Autodesk Fusion 360 part; units mm, degrees
note: some values were not read from the file. Set by a fixed rule: which face or edge a step refers to.
(part 12 of 13)
  spline S4 degree 5 poles (-1.3295, -6.4954) (-1.3295, -6.4955) (-1.3295, -6.4957) (-1.3296, -6.4961) (-1.3297, -6.4966) (-1.3299, -6.4975) (-1.33, -6.4984) (-1.3302, -6.4995) (-1.3304, -6.5007) (-1.3306, -6.502) (-1.3308, -6.5035) (-1.3311, -6.5051) (-1.3313, -6.5068) (-1.3316, -6.5086) (-1.3318, -6.5105) (-1.3321, -6.5126) (-1.3324, -6.5147) (-1.3326, -6.517) (-1.3329, -6.5194) (-1.3332, -6.5219) (-1.3335, -6.5245) (-1.3338, -6.5272) (-1.3341, -6.53) (-1.3343, -6.5329) (-1.3346, -6.5359) (-1.3349, -6.5391) (-1.3352, -6.5423) (-1.3354, -6.5456) (-1.3357, -6.549) (-1.3359, -6.5526) (-1.3362, -6.5562) (-1.3364, -6.5599) (-1.3366, -6.5637) (-1.3368, -6.5676) (-1.337, -6.5716) (-1.3372, -6.5757) (-1.3374, -6.5799) (-1.3376, -6.5842) (-1.3377, -6.5885) (-1.3379, -6.593) (-1.338, -6.5975) (-1.3381, -6.6021) (-1.3382, -6.6069) (-1.3383, -6.6117) (-1.3383, -6.6165) (-1.3384, -6.6215) (-1.3384, -6.6265) (-1.3384, -6.6317) (-1.3384, -6.6369) (-1.3383, -6.6422) (-1.3383, -6.6475) (-1.3382, -6.653) (-1.3381, -6.6585) (-1.338, -6.6641) (-1.3378, -6.6698) (-1.3376, -6.6755) (-1.3374, -6.6814) (-1.3372, -6.6873) (-1.337, -6.6933) (-1.3367, -6.6993) (-1.3364, -6.7054) (-1.3361, -6.7116) (-1.3357, -6.7179) (-1.3353, -6.7242) (-1.3349, -6.7306) (-1.3345, -6.7371) (-1.334, -6.7437) (-1.3335, -6.7503) (-1.333, -6.7569) (-1.3325, -6.7637) (-1.3319, -6.7705) (-1.3313, -6.7774) (-1.3306, -6.7843) (-1.3299, -6.7913) (-1.3292, -6.7984) (-1.3285, -6.8055) (-1.3277, -6.8127) (-1.3269, -6.82) (-1.3261, -6.8273) (-1.3252, -6.8347) (-1.3243, -6.8421) (-1.3234, -6.8496) (-1.3224, -6.8572) (-1.3214, -6.8648) (-1.3204, -6.8725) (-1.3193, -6.8802) (-1.3182, -6.888) (-1.317, -6.8958) (-1.3159, -6.9037) (-1.3146, -6.9117) (-1.3134, -6.9197) (-1.3121, -6.9278) (-1.3108, -6.9359) (-1.3094, -6.9441) (-1.308, -6.9523) (-1.3066, -6.9606) (-1.3051, -6.9689) (-1.3036, -6.9773) (-1.302, -6.9857) (-1.3004, -6.9942) (-1.2988, -7.0027) (-1.2971, -7.0113) (-1.2954, -7.0199) (-1.2936, -7.0286) (-1.2918, -7.0374) (-1.29, -7.0461) (-1.2881, -7.055) (-1.2862, -7.0638) (-1.2843, -7.0728) (-1.2823, -7.0817) (-1.2802, -7.0907) (-1.2782, -7.0998) (-1.276, -7.1089) (-1.2739, -7.118) (-1.2717, -7.1272) (-1.2694, -7.1365) (-1.2671, -7.1457) (-1.2648, -7.1551) (-1.2624, -7.1644) (-1.26, -7.1738) (-1.2575, -7.1833) (-1.255, -7.1928) (-1.2525, -7.2023) (-1.2499, -7.2118) (-1.2473, -7.2215) (-1.2446, -7.2311) (-1.2419, -7.2408) (-1.2391, -7.2505) (-1.2363, -7.2603) (-1.2334, -7.2701) (-1.2305, -7.2799) (-1.2276, -7.2898) (-1.2246, -7.2997) (-1.2215, -7.3096) (-1.2185, -7.3196) (-1.2153, -7.3296) (-1.2122, -7.3397) (-1.2089, -7.3498) (-1.2057, -7.3599) (-1.2024, -7.3701) (-1.199, -7.3803) (-1.1956, -7.3905) (-1.1922, -7.4007) (-1.1887, -7.411) (-1.1851, -7.4214) (-1.1815, -7.4317) (-1.1779, -7.4421) (-1.1742, -7.4525) (-1.1705, -7.463) (-1.1667, -7.4734) (-1.1629, -7.4839) (-1.159, -7.4945) (-1.1551, -7.5051) (-1.1511, -7.5157) (-1.1471, -7.5263) (-1.143, -7.5369) (-1.1389, -7.5476) (-1.1348, -7.5583) (-1.1306, -7.5691) (-1.1263, -7.5798) (-1.122, -7.5906) (-1.1176, -7.6014) (-1.1132, -7.6123) (-1.1088, -7.6232) (-1.1043, -7.6341) (-1.0997, -7.645) (-1.0951, -7.6559) (-1.0905, -7.6669) (-1.0858, -7.6779) (-1.0811, -7.6889) (-1.0763, -7.7) (-1.0714, -7.711) (-1.0665, -7.7221) (-1.0616, -7.7332) (-1.0566, -7.7444) (-1.0516, -7.7555) (-1.0465, -7.7667) (-1.0414, -7.7779) (-1.0362, -7.7891) (-1.0309, -7.8003) (-1.0256, -7.8116) (-1.0203, -7.8229) (-1.0149, -7.8342) (-1.0095, -7.8455) (-1.004, -7.8569) (-0.9985, -7.8682) (-0.9929, -7.8796) (-0.9872, -7.891) (-0.9815, -7.9024) (-0.9758, -7.9138) (-0.97, -7.9253) (-0.9642, -7.9368) (-0.9583, -7.9482) (-0.9524, -7.9597) (-0.9464, -7.9713) (-0.9403, -7.9828) (-0.9342, -7.9943) (-0.9281, -8.0059) (-0.9219, -8.0175) (-0.9157, -8.0291) (-0.9094, -8.0407) (-0.903, -8.0523) (-0.8966, -8.064) (-0.8902, -8.0756) (-0.8837, -8.0873) (-0.8771, -8.099) (-0.8705, -8.1107) (-0.8639, -8.1224) (-0.8572, -8.1341) (-0.8504, -8.1458) (-0.8436, -8.1575) (-0.8368, -8.1693) (-0.8299, -8.1811) (-0.8229, -8.1928) (-0.8159, -8.2046) (-0.8089, -8.2164) (-0.8018, -8.2282) (-0.7946, -8.2401) (-0.7874, -8.2519) (-0.7801, -8.2637) (-0.7728, -8.2756) (-0.7655, -8.2874) (-0.758, -8.2993) (-0.7506, -8.3112) (-0.743, -8.3231) (-0.7355, -8.3349) (-0.7279, -8.3468) (-0.7202, -8.3587) (-0.7125, -8.3707) (-0.7047, -8.3826) (-0.6969, -8.3945) (-0.689, -8.4064) (-0.6811, -8.4184) (-0.6731, -8.4303) (-0.665, -8.4423) (-0.657, -8.4542) (-0.6488, -8.4662) (-0.6406, -8.4782) (-0.6324, -8.4901) (-0.6241, -8.5021) (-0.6158, -8.5141) (-0.6091, -8.5237) (-0.604, -8.5309) (-0.6006, -8.5357) (-0.5989, -8.5381) knots 0 0 0 0 0 0 0.00416667 0.00833333 0.0125 0.01666667 0.02083333 0.025 0.02916667 0.03333333 0.0375 0.04166667 0.04583333 0.05 0.05416667 0.05833333 0.0625 0.06666667 0.07083333 0.075 0.07916667 0.08333333 0.0875 0.09166667 0.09583333 0.1 0.10416667 0.10833333 0.1125 0.11666667 0.12083333 0.125 0.12916667 0.13333333 0.1375 0.14166667 0.14583333 0.15 0.15416667 0.15833333 0.1625 0.16666667 0.17083333 0.175 0.17916667 0.18333333 0.1875 0.19166667 0.19583333 0.2 0.20416667 0.20833333 0.2125 0.21666667 0.22083333 0.225 0.22916667 0.23333333 0.2375 0.24166667 0.24583333 0.25 0.25416667 0.25833333 0.2625 0.26666667 0.27083333 0.275 0.27916667 0.28333333 0.2875 0.29166667 0.29583333 0.3 0.30416667 0.30833333 0.3125 0.31666667 0.32083333 0.325 0.32916667 0.33333333 0.3375 0.34166667 0.34583333 0.35 0.35416667 0.35833333 0.3625 0.36666667 0.37083333 0.375 0.37916667 0.38333333 0.3875 0.39166667 0.39583333 0.4 0.40416667 0.40833333 0.4125 0.41666667 0.42083333 0.425 0.42916667 0.43333333 0.4375 0.44166667 0.44583333 0.45 0.45416667 0.45833333 0.4625 0.46666667 0.47083333 0.475 0.47916667 0.48333333 0.4875 0.49166667 0.49583333 0.5 0.50416667 0.50833333 0.5125 0.51666667 0.52083333 0.525 0.52916667 0.53333333 0.5375 0.54166667 0.54583333 0.55 0.55416667 0.55833333 0.5625 0.56666667 0.57083333 0.575 0.57916667 0.58333333 0.5875 0.59166667 0.59583333 0.6 0.60416667 0.60833333 0.6125 0.61666667 0.62083333 0.625 0.62916667 0.63333333 0.6375 0.64166667 0.64583333 0.65 0.65416667 0.65833333 0.6625 0.66666667 0.67083333 0.675 0.67916667 0.68333333 0.6875 0.69166667 0.69583333 0.7 0.70416667 0.70833333 0.7125 0.71666667 0.72083333 0.725 0.72916667 0.73333333 0.7375 0.74166667 0.74583333 0.75 0.75416667 0.75833333 0.7625 0.76666667 0.77083333 0.775 0.77916667 0.78333333 0.7875 0.79166667 0.79583333 0.8 0.80416667 0.80833333 0.8125 0.81666667 0.82083333 0.825 0.82916667 0.83333333 0.8375 0.84166667 0.84583333 0.85 0.85416667 0.85833333 0.8625 0.86666667 0.87083333 0.875 0.87916667 0.88333333 0.8875 0.89166667 0.89583333 0.9 0.90416667 0.90833333 0.9125 0.91666667 0.92083333 0.925 0.92916667 0.93333333 0.9375 0.94166667 0.94583333 0.95 0.95416667 0.95833333 0.9625 0.96666667 0.97083333 0.975 0.97916667 0.98333333 0.9875 0.99166667 0.99583333 1 1 1 1 1 1
  arc A5 (-0.5989, -8.5381) -> (0.5989, -8.5381) centre (0, 0) ccw
  spline S5 degree 5 poles (0.5989, -8.5381) (0.6006, -8.5357) (0.604, -8.5309) (0.6091, -8.5237) (0.6158, -8.5141) (0.6241, -8.5021) (0.6324, -8.4901) (0.6406, -8.4782) (0.6488, -8.4662) (0.657, -8.4542) (0.665, -8.4423) (0.6731, -8.4303) (0.6811, -8.4184) (0.689, -8.4064) (0.6969, -8.3945) (0.7047, -8.3826) (0.7125, -8.3707) (0.7202, -8.3587) (0.7279, -8.3468) (0.7355, -8.3349) (0.743, -8.3231) (0.7506, -8.3112) (0.758, -8.2993) (0.7655, -8.2874) (0.7728, -8.2756) (0.7801, -8.2637) (0.7874, -8.2519) (0.7946, -8.2401) (0.8018, -8.2282) (0.8089, -8.2164) (0.8159, -8.2046) (0.8229, -8.1928) (0.8299, -8.1811) (0.8368, -8.1693) (0.8436, -8.1575) (0.8504, -8.1458) (0.8572, -8.1341) (0.8639, -8.1224) (0.8705, -8.1107) (0.8771, -8.099) (0.8837, -8.0873) (0.8902, -8.0756) (0.8966, -8.064) (0.903, -8.0523) (0.9094, -8.0407) (0.9157, -8.0291) (0.9219, -8.0175) (0.9281, -8.0059) (0.9342, -7.9943) (0.9403, -7.9828) (0.9464, -7.9713) (0.9524, -7.9597) (0.9583, -7.9482) (0.9642, -7.9368) (0.97, -7.9253) (0.9758, -7.9138) (0.9815, -7.9024) (0.9872, -7.891) (0.9929, -7.8796) (0.9985, -7.8682) (1.004, -7.8569) (1.0095, -7.8455) (1.0149, -7.8342) (1.0203, -7.8229) (1.0256, -7.8116) (1.0309, -7.8003) (1.0362, -7.7891) (1.0414, -7.7779) (1.0465, -7.7667) (1.0516, -7.7555) (1.0566, -7.7444) (1.0616, -7.7332) (1.0665, -7.7221) (1.0714, -7.711) (1.0763, -7.7) (1.0811, -7.6889) (1.0858, -7.6779) (1.0905, -7.6669) (1.0951, -7.6559) (1.0997, -7.645) (1.1043, -7.6341) (1.1088, -7.6232) (1.1132, -7.6123) (1.1176, -7.6014) (1.122, -7.5906) (1.1263, -7.5798) (1.1306, -7.5691) (1.1348, -7.5583) (1.1389, -7.5476) (1.143, -7.5369) (1.1471, -7.5263) (1.1511, -7.5157) (1.1551, -7.5051) (1.159, -7.4945) (1.1629, -7.4839) (1.1667, -7.4734) (1.1705, -7.463) (1.1742, -7.4525) (1.1779, -7.4421) (1.1815, -7.4317) (1.1851, -7.4214) (1.1887, -7.411) (1.1922, -7.4007) (1.1956, -7.3905) (1.199, -7.3803) (1.2024, -7.3701) (1.2057, -7.3599) (1.2089, -7.3498) (1.2122, -7.3397) (1.2153, -7.3296) (1.2185, -7.3196) (1.2215, -7.3096) (1.2246, -7.2997) (1.2276, -7.2898) (1.2305, -7.2799) (1.2334, -7.2701) (1.2363, -7.2603) (1.2391, -7.2505) (1.2419, -7.2408) (1.2446, -7.2311) (1.2473, -7.2215) (1.2499, -7.2118) (1.2525, -7.2023) (1.255, -7.1928) (1.2575, -7.1833) (1.26, -7.1738) (1.2624, -7.1644) (1.2648, -7.1551) (1.2671, -7.1457) (1.2694, -7.1365) (1.2717, -7.1272) (1.2739, -7.118) (1.276, -7.1089) (1.2782, -7.0998) (1.2802, -7.0907) (1.2823, -7.0817) (1.2843, -7.0728) (1.2862, -7.0638) (1.2881, -7.055) (1.29, -7.0461) (1.2918, -7.0374) (1.2936, -7.0286) (1.2954, -7.0199) (1.2971, -7.0113) (1.2988, -7.0027) (1.3004, -6.9942) (1.302, -6.9857) (1.3036, -6.9773) (1.3051, -6.9689) (1.3066, -6.9606) (1.308, -6.9523) (1.3094, -6.9441) (1.3108, -6.9359) (1.3121, -6.9278) (1.3134, -6.9197) (1.3146, -6.9117) (1.3159, -6.9037) (1.317, -6.8958) (1.3182, -6.888) (1.3193, -6.8802) (1.3204, -6.8725) (1.3214, -6.8648) (1.3224, -6.8572) (1.3234, -6.8496) (1.3243, -6.8421) (1.3252, -6.8347) (1.3261, -6.8273) (1.3269, -6.82) (1.3277, -6.8127) (1.3285, -6.8055) (1.3292, -6.7984) (1.3299, -6.7913) (1.3306, -6.7843) (1.3313, -6.7774) (1.3319, -6.7705) (1.3325, -6.7637) (1.333, -6.7569) (1.3335, -6.7503) (1.334, -6.7437) (1.3345, -6.7371) (1.3349, -6.7306) (1.3353, -6.7242) (1.3357, -6.7179) (1.3361, -6.7116) (1.3364, -6.7054) (1.3367, -6.6993) (1.337, -6.6933) (1.3372, -6.6873) (1.3374, -6.6814) (1.3376, -6.6755) (1.3378, -6.6698) (1.338, -6.6641) (1.3381, -6.6585) (1.3382, -6.653) (1.3383, -6.6475) (1.3383, -6.6422) (1.3384, -6.6369) (1.3384, -6.6317) (1.3384, -6.6265) (1.3384, -6.6215) (1.3383, -6.6165) (1.3383, -6.6117) (1.3382, -6.6069) (1.3381, -6.6021) (1.338, -6.5975) (1.3379, -6.593) (1.3377, -6.5885) (1.3376, -6.5842) (1.3374, -6.5799) (1.3372, -6.5757) (1.337, -6.5716) (1.3368, -6.5676) (1.3366, -6.5637) (1.3364, -6.5599) (1.3362, -6.5562) (1.3359, -6.5526) (1.3357, -6.549) (1.3354, -6.5456) (1.3352, -6.5423) (1.3349, -6.5391) (1.3346, -6.5359) (1.3343, -6.5329) (1.3341, -6.53) (1.3338, -6.5272) (1.3335, -6.5245) (1.3332, -6.5219) (1.3329, -6.5194) (1.3326, -6.517) (1.3324, -6.5147) (1.3321, -6.5126) (1.3318, -6.5105) (1.3316, -6.5086) (1.3313, -6.5068) (1.3311, -6.5051) (1.3308, -6.5035) (1.3306, -6.502) (1.3304, -6.5007) (1.3302, -6.4995) (1.33, -6.4984) (1.3299, -6.4975) (1.3297, -6.4966) (1.3296, -6.4961) (1.3295, -6.4957) (1.3295, -6.4955) (1.3295, -6.4954) knots -1 -1 -1 -1 -1 -1 -0.99583333 -0.99166667 -0.9875 -0.98333333 -0.97916667 -0.975 -0.97083333 -0.96666667 -0.9625 -0.95833333 -0.95416667 -0.95 -0.94583333 -0.94166667 -0.9375 -0.93333333 -0.92916667 -0.925 -0.92083333 -0.91666667 -0.9125 -0.90833333 -0.90416667 -0.9 -0.89583333 -0.89166667 -0.8875 -0.88333333 -0.87916667 -0.875 -0.87083333 -0.86666667 -0.8625 -0.85833333 -0.85416667 -0.85 -0.84583333 -0.84166667 -0.8375 -0.83333333 -0.82916667 -0.825 -0.82083333 -0.81666667 -0.8125 -0.80833333 -0.80416667 -0.8 -0.79583333 -0.79166667 -0.7875 -0.78333333 -0.77916667 -0.775 -0.77083333 -0.76666667 -0.7625 -0.75833333 -0.75416667 -0.75 -0.74583333 -0.74166667 -0.7375 -0.73333333 -0.72916667 -0.725 -0.72083333 -0.71666667 -0.7125 -0.70833333 -0.70416667 -0.7 -0.69583333 -0.69166667 -0.6875 -0.68333333 -0.67916667 -0.675 -0.67083333 -0.66666667 -0.6625 -0.65833333 -0.65416667 -0.65 -0.64583333 -0.64166667 -0.6375 -0.63333333 -0.62916667 -0.625 -0.62083333 -0.61666667 -0.6125 -0.60833333 -0.60416667 -0.6 -0.59583333 -0.59166667 -0.5875 -0.58333333 -0.57916667 -0.575 -0.57083333 -0.56666667 -0.5625 -0.55833333 -0.55416667 -0.55 -0.54583333 -0.54166667 -0.5375 -0.53333333 -0.52916667 -0.525 -0.52083333 -0.51666667 -0.5125 -0.50833333 -0.50416667 -0.5 -0.49583333 -0.49166667 -0.4875 -0.48333333 -0.47916667 -0.475 -0.47083333 -0.46666667 -0.4625 -0.45833333 -0.45416667 -0.45 -0.44583333 -0.44166667 -0.4375 -0.43333333 -0.42916667 -0.425 -0.42083333 -0.41666667 -0.4125 -0.40833333 -0.40416667 -0.4 -0.39583333 -0.39166667 -0.3875 -0.38333333 -0.37916667 -0.375 -0.37083333 -0.36666667 -0.3625 -0.35833333 -0.35416667 -0.35 -0.34583333 -0.34166667 -0.3375 -0.33333333 -0.32916667 -0.325 -0.32083333 -0.31666667 -0.3125 -0.30833333 -0.30416667 -0.3 -0.29583333 -0.29166667 -0.2875 -0.28333333 -0.27916667 -0.275 -0.27083333 -0.26666667 -0.2625 -0.25833333 -0.25416667 -0.25 -0.24583333 -0.24166667 -0.2375 -0.23333333 -0.22916667 -0.225 -0.22083333 -0.21666667 -0.2125 -0.20833333 -0.20416667 -0.2 -0.19583333 -0.19166667 -0.1875 -0.18333333 -0.17916667 -0.175 -0.17083333 -0.16666667 -0.1625 -0.15833333 -0.15416667 -0.15 -0.14583333 -0.14166667 -0.1375 -0.13333333 -0.12916667 -0.125 -0.12083333 -0.11666667 -0.1125 -0.10833333 -0.10416667 -0.1 -0.09583333 -0.09166667 -0.0875 -0.08333333 -0.07916667 -0.075 -0.07083333 -0.06666667 -0.0625 -0.05833333 -0.05416667 -0.05 -0.04583333 -0.04166667 -0.0375 -0.03333333 -0.02916667 -0.025 -0.02083333 -0.01666667 -0.0125 -0.00833333 -0.00416667 0 0 0 0 0 0
  line L10 (1.3295, -6.4954) -> (1.3293, -6.4945)
  line L11 (1.3293, -6.4945) -> (0.944, -4.6119)
  arc A6 (0.944, -4.6119) -> (2.5936, -3.9286) centre (0, 0) ccw
  line L12 (2.5936, -3.9286) -> (3.6523, -5.5323)
  line L13 (3.6523, -5.5323) -> (3.6529, -5.533)
  spline S6 degree 5 poles (3.6529, -5.533) (3.6529, -5.5331) (3.653, -5.5333) (3.6532, -5.5336) (3.6536, -5.5341) (3.654, -5.5348) (3.6546, -5.5355) (3.6552, -5.5364) (3.656, -5.5374) (3.6568, -5.5385) (3.6576, -5.5397) (3.6586, -5.541) (3.6596, -5.5424) (3.6607, -5.5438) (3.6619, -5.5454) (3.6632, -5.547) (3.6645, -5.5487) (3.6659, -5.5505) (3.6674, -5.5524) (3.6689, -5.5544) (3.6706, -5.5564) (3.6723, -5.5585) (3.6741, -5.5607) (3.676, -5.563) (3.6779, -5.5653) (3.6799, -5.5677) (3.682, -5.5702) (3.6842, -5.5727) (3.6864, -5.5753) (3.6887, -5.578) (3.6911, -5.5807) (3.6936, -5.5835) (3.6961, -5.5864) (3.6987, -5.5893) (3.7014, -5.5923) (3.7042, -5.5953) (3.707, -5.5984) (3.7099, -5.6015) (3.7129, -5.6047) (3.7159, -5.608) (3.719, -5.6113) (3.7222, -5.6146) (3.7255, -5.618) (3.7288, -5.6214) (3.7323, -5.6249) (3.7357, -5.6285) (3.7393, -5.6321) (3.7429, -5.6357) (3.7466, -5.6394) (3.7504, -5.6431) (3.7542, -5.6468) (3.7581, -5.6506) (3.7621, -5.6544) (3.7662, -5.6583) (3.7703, -5.6622) (3.7745, -5.6662) (3.7787, -5.6702) (3.7831, -5.6742) (3.7875, -5.6782) (3.7919, -5.6823) (3.7965, -5.6864) (3.8011, -5.6906) (3.8058, -5.6948) (3.8105, -5.699) (3.8153, -5.7032) (3.8202, -5.7075) (3.8252, -5.7118) (3.8302, -5.7161) (3.8353, -5.7205) (3.8405, -5.7248) (3.8457, -5.7292) (3.851, -5.7337) (3.8563, -5.7381) (3.8618, -5.7426) (3.8673, -5.7471) (3.8728, -5.7516) (3.8785, -5.7562) (3.8842, -5.7607) (3.8899, -5.7653) (3.8958, -5.7699) (3.9017, -5.7745) (3.9076, -5.7792) (3.9137, -5.7838) (3.9198, -5.7885) (3.9259, -5.7932) (3.9321, -5.7979) (3.9384, -5.8026) (3.9448, -5.8074) (3.9512, -5.8121) (3.9577, -5.8169) (3.9643, -5.8217) (3.9709, -5.8265) (3.9776, -5.8313) (3.9843, -5.8361) (3.9911, -5.8409) (3.998, -5.8457) (4.0049, -5.8506) (4.0119, -5.8554) (4.019, -5.8603) (4.0261, -5.8652) (4.0333, -5.8701) (4.0406, -5.8749) (4.0479, -5.8798) (4.0553, -5.8847) (4.0627, -5.8896) (4.0702, -5.8945) (4.0778, -5.8995) (4.0854, -5.9044) (4.0931, -5.9093) (4.1008, -5.9142) (4.1086, -5.9192) (4.1165, -5.9241) (4.1245, -5.929) (4.1325, -5.934) (4.1405, -5.9389) (4.1486, -5.9439) (4.1568, -5.9488) (4.165, -5.9537) (4.1733, -5.9587) (4.1817, -5.9636) (4.1901, -5.9686) (4.1986, -5.9735) (4.2071, -5.9784) (4.2157, -5.9834) (4.2244, -5.9883) (4.2331, -5.9932) (4.2419, -5.9981) (4.2507, -6.0031) (4.2596, -6.008) (4.2686, -6.0129) (4.2776, -6.0178) (4.2866, -6.0227) (4.2958, -6.0276) (4.3049, -6.0325) (4.3142, -6.0373) (4.3235, -6.0422) (4.3328, -6.0471) (4.3422, -6.0519) (4.3517, -6.0568) (4.3612, -6.0616) (4.3708, -6.0665) (4.3804, -6.0713) (4.3901, -6.0761) (4.3999, -6.0809) (4.4097, -6.0857) (4.4195, -6.0905) (4.4295, -6.0952) (4.4394, -6.1) (4.4495, -6.1048) (4.4595, -6.1095) (4.4697, -6.1142) (4.4799, -6.1189) (4.4901, -6.1236) (4.5004, -6.1283) (4.5108, -6.133) (4.5212, -6.1377) (4.5316, -6.1423) (4.5421, -6.1469) (4.5527, -6.1516) (4.5633, -6.1562) (4.574, -6.1607) (4.5847, -6.1653) (4.5955, -6.1699) (4.6064, -6.1744) (4.6172, -6.1789) (4.6282, -6.1835) (4.6392, -6.1879) (4.6502, -6.1924) (4.6613, -6.1969) (4.6725, -6.2013) (4.6836, -6.2057) (4.6949, -6.2101) (4.7062, -6.2145) (4.7175, -6.2189) (4.7289, -6.2232) (4.7404, -6.2275) (4.7519, -6.2319) (4.7634, -6.2361) (4.7751, -6.2404) (4.7867, -6.2447) (4.7984, -6.2489) (4.8102, -6.2531) (4.822, -6.2573) (4.8338, -6.2614) (4.8457, -6.2656) (4.8577, -6.2697) (4.8696, -6.2738) (4.8817, -6.2779) (4.8938, -6.2819) (4.9059, -6.2859) (4.9181, -6.2899) (4.9304, -6.2939) (4.9426, -6.2979) (4.955, -6.3018) (4.9673, -6.3057) (4.9798, -6.3096) (4.9922, -6.3135) (5.0048, -6.3173) (5.0173, -6.3211) (5.0299, -6.3249) (5.0426, -6.3287) (5.0553, -6.3324) (5.0681, -6.3361) (5.0809, -6.3398) (5.0937, -6.3434) (5.1066, -6.3471) (5.1195, -6.3507) (5.1325, -6.3542) (5.1455, -6.3578) (5.1586, -6.3613) (5.1717, -6.3648) (5.1849, -6.3683) (5.1981, -6.3717) (5.2113, -6.3751) (5.2246, -6.3785) (5.2379, -6.3819) (5.2513, -6.3852) (5.2647, -6.3885) (5.2782, -6.3917) (5.2917, -6.395) (5.3053, -6.3982) (5.3188, -6.4014) (5.3325, -6.4045) (5.3462, -6.4076) (5.3599, -6.4107) (5.3736, -6.4138) (5.3874, -6.4168) (5.4013, -6.4198) (5.4152, -6.4227) (5.4291, -6.4257) (5.4431, -6.4286) (5.4571, -6.4314) (5.4711, -6.4343) (5.4852, -6.4371) (5.4993, -6.4399) (5.5135, -6.4426) (5.5277, -6.4453) (5.542, -6.448) (5.5563, -6.4506) (5.5706, -6.4532) (5.585, -6.4558) (5.5965, -6.4578) (5.6051, -6.4593) (5.6109, -6.4603) (5.6138, -6.4608) knots 0 0 0 0 0 0 0.00416667 0.00833333 0.0125 0.01666667 0.02083333 0.025 0.02916667 0.03333333 0.0375 0.04166667 0.04583333 0.05 0.05416667 0.05833333 0.0625 0.06666667 0.07083333 0.075 0.07916667 0.08333333 0.0875 0.09166667 0.09583333 0.1 0.10416667 0.10833333 0.1125 0.11666667 0.12083333 0.125 0.12916667 0.13333333 0.1375 0.14166667 0.14583333 0.15 0.15416667 0.15833333 0.1625 0.16666667 0.17083333 0.175 0.17916667 0.18333333 0.1875 0.19166667 0.19583333 0.2 0.20416667 0.20833333 0.2125 0.21666667 0.22083333 0.225 0.22916667 0.23333333 0.2375 0.24166667 0.24583333 0.25 0.25416667 0.25833333 0.2625 0.26666667 0.27083333 0.275 0.27916667 0.28333333 0.2875 0.29166667 0.29583333 0.3 0.30416667 0.30833333 0.3125 0.31666667 0.32083333 0.325 0.32916667 0.33333333 0.3375 0.34166667 0.34583333 0.35 0.35416667 0.35833333 0.3625 0.36666667 0.37083333 0.375 0.37916667 0.38333333 0.3875 0.39166667 0.39583333 0.4 0.40416667 0.40833333 0.4125 0.41666667 0.42083333 0.425 0.42916667 0.43333333 0.4375 0.44166667 0.44583333 0.45 0.45416667 0.45833333 0.4625 0.46666667 0.47083333 0.475 0.47916667 0.48333333 0.4875 0.49166667 0.49583333 0.5 0.50416667 0.50833333 0.5125 0.51666667 0.52083333 0.525 0.52916667 0.53333333 0.5375 0.54166667 0.54583333 0.55 0.55416667 0.55833333 0.5625 0.56666667 0.57083333 0.575 0.57916667 0.58333333 0.5875 0.59166667 0.59583333 0.6 0.60416667 0.60833333 0.6125 0.61666667 0.62083333 0.625 0.62916667 0.63333333 0.6375 0.64166667 0.64583333 0.65 0.65416667 0.65833333 0.6625 0.66666667 0.67083333 0.675 0.67916667 0.68333333 0.6875 0.69166667 0.69583333 0.7 0.70416667 0.70833333 0.7125 0.71666667 0.72083333 0.725 0.72916667 0.73333333 0.7375 0.74166667 0.74583333 0.75 0.75416667 0.75833333 0.7625 0.76666667 0.77083333 0.775 0.77916667 0.78333333 0.7875 0.79166667 0.79583333 0.8 0.80416667 0.80833333 0.8125 0.81666667 0.82083333 0.825 0.82916667 0.83333333 0.8375 0.84166667 0.84583333 0.85 0.85416667 0.85833333 0.8625 0.86666667 0.87083333 0.875 0.87916667 0.88333333 0.8875 0.89166667 0.89583333 0.9 0.90416667 0.90833333 0.9125 0.91666667 0.92083333 0.925 0.92916667 0.93333333 0.9375 0.94166667 0.94583333 0.95 0.95416667 0.95833333 0.9625 0.96666667 0.97083333 0.975 0.97916667 0.98333333 0.9875 0.99166667 0.99583333 1 1 1 1 1 1
  arc A7 (5.6138, -6.4608) -> (6.4608, -5.6138) centre (0, 0) ccw
  spline S7 degree 5 poles (6.4608, -5.6138) (6.4603, -5.6109) (6.4593, -5.6051) (6.4578, -5.5965) (6.4558, -5.585) (6.4532, -5.5706) (6.4506, -5.5563) (6.448, -5.542) (6.4453, -5.5277) (6.4426, -5.5135) (6.4399, -5.4993) (6.4371, -5.4852) (6.4343, -5.4711) (6.4314, -5.4571) (6.4286, -5.4431) (6.4257, -5.4291) (6.4227, -5.4152) (6.4198, -5.4013) (6.4168, -5.3874) (6.4138, -5.3736) (6.4107, -5.3599) (6.4076, -5.3462) (6.4045, -5.3325) (6.4014, -5.3188) (6.3982, -5.3053) (6.395, -5.2917) (6.3917, -5.2782) (6.3885, -5.2647) (6.3852, -5.2513) (6.3819, -5.2379) (6.3785, -5.2246) (6.3751, -5.2113) (6.3717, -5.1981) (6.3683, -5.1849) (6.3648, -5.1717) (6.3613, -5.1586) (6.3578, -5.1455) (6.3542, -5.1325) (6.3507, -5.1195) (6.3471, -5.1066) (6.3434, -5.0937) (6.3398, -5.0809) (6.3361, -5.0681) (6.3324, -5.0553) (6.3287, -5.0426) (6.3249, -5.0299) (6.3211, -5.0173) (6.3173, -5.0048) (6.3135, -4.9922) (6.3096, -4.9798) (6.3057, -4.9673) (6.3018, -4.955) (6.2979, -4.9426) (6.2939, -4.9304) (6.2899, -4.9181) (6.2859, -4.9059) (6.2819, -4.8938) (6.2779, -4.8817) (6.2738, -4.8696) (6.2697, -4.8577) (6.2656, -4.8457) (6.2614, -4.8338) (6.2573, -4.822) (6.2531, -4.8102) (6.2489, -4.7984) (6.2447, -4.7867) (6.2404, -4.7751) (6.2361, -4.7634) (6.2319, -4.7519) (6.2275, -4.7404) (6.2232, -4.7289) (6.2189, -4.7175) (6.2145, -4.7062) (6.2101, -4.6949) (6.2057, -4.6836) (6.2013, -4.6725) (6.1969, -4.6613) (6.1924, -4.6502) (6.1879, -4.6392) (6.1835, -4.6282) (6.1789, -4.6172) (6.1744, -4.6064) (6.1699, -4.5955) (6.1653, -4.5847) (6.1607, -4.574) (6.1562, -4.5633) (6.1516, -4.5527) (6.1469, -4.5421) (6.1423, -4.5316) (6.1377, -4.5212) (6.133, -4.5108) (6.1283, -4.5004) (6.1236, -4.4901) (6.1189, -4.4799) (6.1142, -4.4697) (6.1095, -4.4595) (6.1048, -4.4495) (6.1, -4.4394) (6.0952, -4.4295) (6.0905, -4.4195) (6.0857, -4.4097) (6.0809, -4.3999) (6.0761, -4.3901) (6.0713, -4.3804) (6.0665, -4.3708) (6.0616, -4.3612) (6.0568, -4.3517) (6.0519, -4.3422) (6.0471, -4.3328) (6.0422, -4.3235) (6.0373, -4.3142) (6.0325, -4.3049) (6.0276, -4.2958) (6.0227, -4.2866) (6.0178, -4.2776) (6.0129, -4.2686) (6.008, -4.2596) (6.0031, -4.2507) (5.9981, -4.2419) (5.9932, -4.2331) (5.9883, -4.2244) (5.9834, -4.2157) (5.9784, -4.2071) (5.9735, -4.1986) (5.9686, -4.1901) (5.9636, -4.1817) (5.9587, -4.1733) (5.9537, -4.165) (5.9488, -4.1568) (5.9439, -4.1486) (5.9389, -4.1405) (5.934, -4.1325) (5.929, -4.1245) (5.9241, -4.1165) (5.9192, -4.1086) (5.9142, -4.1008) (5.9093, -4.0931) (5.9044, -4.0854) (5.8995, -4.0778) (5.8945, -4.0702) (5.8896, -4.0627) (5.8847, -4.0553) (5.8798, -4.0479) (5.8749, -4.0406) (5.8701, -4.0333) (5.8652, -4.0261) (5.8603, -4.019) (5.8554, -4.0119) (5.8506, -4.0049) (5.8457, -3.998) (5.8409, -3.9911) (5.8361, -3.9843) (5.8313, -3.9776) (5.8265, -3.9709) (5.8217, -3.9643) (5.8169, -3.9577) (5.8121, -3.9512) (5.8074, -3.9448) (5.8026, -3.9384) (5.7979, -3.9321) (5.7932, -3.9259) (5.7885, -3.9198) (5.7838, -3.9137) (5.7792, -3.9076) (5.7745, -3.9017) (5.7699, -3.8958) (5.7653, -3.8899) (5.7607, -3.8842) (5.7562, -3.8785) (5.7516, -3.8728) (5.7471, -3.8673) (5.7426, -3.8618) (5.7381, -3.8563) (5.7337, -3.851) (5.7292, -3.8457) (5.7248, -3.8405) (5.7205, -3.8353) (5.7161, -3.8302) (5.7118, -3.8252) (5.7075, -3.8202) (5.7032, -3.8153) (5.699, -3.8105) (5.6948, -3.8058) (5.6906, -3.8011) (5.6864, -3.7965) (5.6823, -3.7919) (5.6782, -3.7875) (5.6742, -3.7831) (5.6702, -3.7787) (5.6662, -3.7745) (5.6622, -3.7703) (5.6583, -3.7662) (5.6544, -3.7621) (5.6506, -3.7581) (5.6468, -3.7542) (5.6431, -3.7504) (5.6394, -3.7466) (5.6357, -3.7429) (5.6321, -3.7393) (5.6285, -3.7357) (5.6249, -3.7323) (5.6214, -3.7288) (5.618, -3.7255) (5.6146, -3.7222) (5.6113, -3.719) (5.608, -3.7159) (5.6047, -3.7129) (5.6015, -3.7099) (5.5984, -3.707) (5.5953, -3.7042) (5.5923, -3.7014) (5.5893, -3.6987) (5.5864, -3.6961) (5.5835, -3.6936) (5.5807, -3.6911) (5.578, -3.6887) (5.5753, -3.6864) (5.5727, -3.6842) (5.5702, -3.682) (5.5677, -3.6799) (5.5653, -3.6779) (5.563, -3.676) (5.5607, -3.6741) (5.5585, -3.6723) (5.5564, -3.6706) (5.5544, -3.6689) (5.5524, -3.6674) (5.5505, -3.6659) (5.5487, -3.6645) (5.547, -3.6632) (5.5454, -3.6619) (5.5438, -3.6607) (5.5424, -3.6596) (5.541, -3.6586) (5.5397, -3.6576) (5.5385, -3.6568) (5.5374, -3.656) (5.5364, -3.6552) (5.5355, -3.6546) (5.5348, -3.654) (5.5341, -3.6536) (5.5336, -3.6532) (5.5333, -3.653) (5.5331, -3.6529) (5.533, -3.6529) knots -1 -1 -1 -1 -1 -1 -0.99583333 -0.99166667 -0.9875 -0.98333333 -0.97916667 -0.975 -0.97083333 -0.96666667 -0.9625 -0.95833333 -0.95416667 -0.95 -0.94583333 -0.94166667 -0.9375 -0.93333333 -0.92916667 -0.925 -0.92083333 -0.91666667 -0.9125 -0.90833333 -0.90416667 -0.9 -0.89583333 -0.89166667 -0.8875 -0.88333333 -0.87916667 -0.875 -0.87083333 -0.86666667 -0.8625 -0.85833333 -0.85416667 -0.85 -0.84583333 -0.84166667 -0.8375 -0.83333333 -0.82916667 -0.825 -0.82083333 -0.81666667 -0.8125 -0.80833333 -0.80416667 -0.8 -0.79583333 -0.79166667 -0.7875 -0.78333333 -0.77916667 -0.775 -0.77083333 -0.76666667 -0.7625 -0.75833333 -0.75416667 -0.75 -0.74583333 -0.74166667 -0.7375 -0.73333333 -0.72916667 -0.725 -0.72083333 -0.71666667 -0.7125 -0.70833333 -0.70416667 -0.7 -0.69583333 -0.69166667 -0.6875 -0.68333333 -0.67916667 -0.675 -0.67083333 -0.66666667 -0.6625 -0.65833333 -0.65416667 -0.65 -0.64583333 -0.64166667 -0.6375 -0.63333333 -0.62916667 -0.625 -0.62083333 -0.61666667 -0.6125 -0.60833333 -0.60416667 -0.6 -0.59583333 -0.59166667 -0.5875 -0.58333333 -0.57916667 -0.575 -0.57083333 -0.56666667 -0.5625 -0.55833333 -0.55416667 -0.55 -0.54583333 -0.54166667 -0.5375 -0.53333333 -0.52916667 -0.525 -0.52083333 -0.51666667 -0.5125 -0.50833333 -0.50416667 -0.5 -0.49583333 -0.49166667 -0.4875 -0.48333333 -0.47916667 -0.475 -0.47083333 -0.46666667 -0.4625 -0.45833333 -0.45416667 -0.45 -0.44583333 -0.44166667 -0.4375 -0.43333333 -0.42916667 -0.425 -0.42083333 -0.41666667 -0.4125 -0.40833333 -0.40416667 -0.4 -0.39583333 -0.39166667 -0.3875 -0.38333333 -0.37916667 -0.375 -0.37083333 -0.36666667 -0.3625 -0.35833333 -0.35416667 -0.35 -0.34583333 -0.34166667 -0.3375 -0.33333333 -0.32916667 -0.325 -0.32083333 -0.31666667 -0.3125 -0.30833333 -0.30416667 -0.3 -0.29583333 -0.29166667 -0.2875 -0.28333333 -0.27916667 -0.275 -0.27083333 -0.26666667 -0.2625 -0.25833333 -0.25416667 -0.25 -0.24583333 -0.24166667 -0.2375 -0.23333333 -0.22916667 -0.225 -0.22083333 -0.21666667 -0.2125 -0.20833333 -0.20416667 -0.2 -0.19583333 -0.19166667 -0.1875 -0.18333333 -0.17916667 -0.175 -0.17083333 -0.16666667 -0.1625 -0.15833333 -0.15416667 -0.15 -0.14583333 -0.14166667 -0.1375 -0.13333333 -0.12916667 -0.125 -0.12083333 -0.11666667 -0.1125 -0.10833333 -0.10416667 -0.1 -0.09583333 -0.09166667 -0.0875 -0.08333333 -0.07916667 -0.075 -0.07083333 -0.06666667 -0.0625 -0.05833333 -0.05416667 -0.05 -0.04583333 -0.04166667 -0.0375 -0.03333333 -0.02916667 -0.025 -0.02083333 -0.01666667 -0.0125 -0.00833333 -0.00416667 0 0 0 0 0 0
  line L14 (5.533, -3.6529) -> (5.5323, -3.6523)
  line L15 (5.5323, -3.6523) -> (3.9286, -2.5936)
  arc A8 (3.9286, -2.5936) -> (4.6119, -0.944) centre (0, 0) ccw
  line L16 (4.6119, -0.944) -> (6.4945, -1.3293)
  line L17 (6.4945, -1.3293) -> (6.4954, -1.3295)
  spline S8 degree 5 poles (6.4954, -1.3295) (6.4955, -1.3295) (6.4957, -1.3295) (6.4961, -1.3296) (6.4966, -1.3297) (6.4975, -1.3299) (6.4984, -1.33) (6.4995, -1.3302) (6.5007, -1.3304) (6.502, -1.3306) (6.5035, -1.3308) (6.5051, -1.3311) (6.5068, -1.3313) (6.5086, -1.3316) (6.5105, -1.3318) (6.5126, -1.3321) (6.5147, -1.3324) (6.517, -1.3326) (6.5194, -1.3329) (6.5219, -1.3332) (6.5245, -1.3335) (6.5272, -1.3338) (6.53, -1.3341) (6.5329, -1.3343) (6.5359, -1.3346) (6.5391, -1.3349) (6.5423, -1.3352) (6.5456, -1.3354) (6.549, -1.3357) (6.5526, -1.3359) (6.5562, -1.3362) (6.5599, -1.3364) (6.5637, -1.3366) (6.5676, -1.3368) (6.5716, -1.337) (6.5757, -1.3372) (6.5799, -1.3374) (6.5842, -1.3376) (6.5885, -1.3377) (6.593, -1.3379) (6.5975, -1.338) (6.6021, -1.3381) (6.6069, -1.3382) (6.6117, -1.3383) (6.6165, -1.3383) (6.6215, -1.3384) (6.6265, -1.3384) (6.6317, -1.3384) (6.6369, -1.3384) (6.6422, -1.3383) (6.6475, -1.3383) (6.653, -1.3382) (6.6585, -1.3381) (6.6641, -1.338) (6.6698, -1.3378) (6.6755, -1.3376) (6.6814, -1.3374) (6.6873, -1.3372) (6.6933, -1.337) (6.6993, -1.3367) (6.7054, -1.3364) (6.7116, -1.3361) (6.7179, -1.3357) (6.7242, -1.3353) (6.7306, -1.3349) (6.7371, -1.3345) (6.7437, -1.334) (6.7503, -1.3335) (6.7569, -1.333) (6.7637, -1.3325) (6.7705, -1.3319) (6.7774, -1.3313) (6.7843, -1.3306) (6.7913, -1.3299) (6.7984, -1.3292) (6.8055, -1.3285) (6.8127, -1.3277) (6.82, -1.3269) (6.8273, -1.3261) (6.8347, -1.3252) (6.8421, -1.3243) (6.8496, -1.3234) (6.8572, -1.3224) (6.8648, -1.3214) (6.8725, -1.3204) (6.8802, -1.3193) (6.888, -1.3182) (6.8958, -1.317) (6.9037, -1.3159) (6.9117, -1.3146) (6.9197, -1.3134) (6.9278, -1.3121) (6.9359, -1.3108) (6.9441, -1.3094) (6.9523, -1.308) (6.9606, -1.3066) (6.9689, -1.3051) (6.9773, -1.3036) (6.9857, -1.302) (6.9942, -1.3004) (7.0027, -1.2988) (7.0113, -1.2971) (7.0199, -1.2954) (7.0286, -1.2936) (7.0374, -1.2918) (7.0461, -1.29) (7.055, -1.2881) (7.0638, -1.2862) (7.0728, -1.2843) (7.0817, -1.2823) (7.0907, -1.2802) (7.0998, -1.2782) (7.1089, -1.276) (7.118, -1.2739) (7.1272, -1.2717) (7.1365, -1.2694) (7.1457, -1.2671) (7.1551, -1.2648) (7.1644, -1.2624) (7.1738, -1.26) (7.1833, -1.2575) (7.1928, -1.255) (7.2023, -1.2525) (7.2118, -1.2499) (7.2215, -1.2473) (7.2311, -1.2446) (7.2408, -1.2419) (7.2505, -1.2391) (7.2603, -1.2363) (7.2701, -1.2334) (7.2799, -1.2305) (7.2898, -1.2276) (7.2997, -1.2246) (7.3096, -1.2215) (7.3196, -1.2185) (7.3296, -1.2153) (7.3397, -1.2122) (7.3498, -1.2089) (7.3599, -1.2057) (7.3701, -1.2024) (7.3803, -1.199) (7.3905, -1.1956) (7.4007, -1.1922) (7.411, -1.1887) (7.4214, -1.1851) (7.4317, -1.1815) (7.4421, -1.1779) (7.4525, -1.1742) (7.463, -1.1705) (7.4734, -1.1667) (7.4839, -1.1629) (7.4945, -1.159) (7.5051, -1.1551) (7.5157, -1.1511) (7.5263, -1.1471) (7.5369, -1.143) (7.5476, -1.1389) (7.5583, -1.1348) (7.5691, -1.1306) (7.5798, -1.1263) (7.5906, -1.122) (7.6014, -1.1176) (7.6123, -1.1132) (7.6232, -1.1088) (7.6341, -1.1043) (7.645, -1.0997) (7.6559, -1.0951) (7.6669, -1.0905) (7.6779, -1.0858) (7.6889, -1.0811) (7.7, -1.0763) (7.711, -1.0714) (7.7221, -1.0665) (7.7332, -1.0616) (7.7444, -1.0566) (7.7555, -1.0516) (7.7667, -1.0465) (7.7779, -1.0414) (7.7891, -1.0362) (7.8003, -1.0309) (7.8116, -1.0256) (7.8229, -1.0203) (7.8342, -1.0149) (7.8455, -1.0095) (7.8569, -1.004) (7.8682, -0.9985) (7.8796, -0.9929) (7.891, -0.9872) (7.9024, -0.9815) (7.9138, -0.9758) (7.9253, -0.97) (7.9368, -0.9642) (7.9482, -0.9583) (7.9597, -0.9524) (7.9713, -0.9464) (7.9828, -0.9403) (7.9943, -0.9342) (8.0059, -0.9281) (8.0175, -0.9219) (8.0291, -0.9157) (8.0407, -0.9094) (8.0523, -0.903) (8.064, -0.8966) (8.0756, -0.8902) (8.0873, -0.8837) (8.099, -0.8771) (8.1107, -0.8705) (8.1224, -0.8639) (8.1341, -0.8572) (8.1458, -0.8504) (8.1575, -0.8436) (8.1693, -0.8368) (8.1811, -0.8299) (8.1928, -0.8229) (8.2046, -0.8159) (8.2164, -0.8089) (8.2282, -0.8018) (8.2401, -0.7946) (8.2519, -0.7874) (8.2637, -0.7801) (8.2756, -0.7728) (8.2874, -0.7655) (8.2993, -0.758) (8.3112, -0.7506) (8.3231, -0.743) (8.3349, -0.7355) (8.3468, -0.7279) (8.3587, -0.7202) (8.3707, -0.7125) (8.3826, -0.7047) (8.3945, -0.6969) (8.4064, -0.689) (8.4184, -0.6811) (8.4303, -0.6731) (8.4423, -0.665) (8.4542, -0.657) (8.4662, -0.6488) (8.4782, -0.6406) (8.4901, -0.6324) (8.5021, -0.6241) (8.5141, -0.6158) (8.5237, -0.6091) (8.5309, -0.604) (8.5357, -0.6006) (8.5381, -0.5989) knots 0 0 0 0 0 0 0.00416667 0.00833333 0.0125 0.01666667 0.02083333 0.025 0.02916667 0.03333333 0.0375 0.04166667 0.04583333 0.05 0.05416667 0.05833333 0.0625 0.06666667 0.07083333 0.075 0.07916667 0.08333333 0.0875 0.09166667 0.09583333 0.1 0.10416667 0.10833333 0.1125 0.11666667 0.12083333 0.125 0.12916667 0.13333333 0.1375 0.14166667 0.14583333 0.15 0.15416667 0.15833333 0.1625 0.16666667 0.17083333 0.175 0.17916667 0.18333333 0.1875 0.19166667 0.19583333 0.2 0.20416667 0.20833333 0.2125 0.21666667 0.22083333 0.225 0.22916667 0.23333333 0.2375 0.24166667 0.24583333 0.25 0.25416667 0.25833333 0.2625 0.26666667 0.27083333 0.275 0.27916667 0.28333333 0.2875 0.29166667 0.29583333 0.3 0.30416667 0.30833333 0.3125 0.31666667 0.32083333 0.325 0.32916667 0.33333333 0.3375 0.34166667 0.34583333 0.35 0.35416667 0.35833333 0.3625 0.36666667 0.37083333 0.375 0.37916667 0.38333333 0.3875 0.39166667 0.39583333 0.4 0.40416667 0.40833333 0.4125 0.41666667 0.42083333 0.425 0.42916667 0.43333333 0.4375 0.44166667 0.44583333 0.45 0.45416667 0.45833333 0.4625 0.46666667 0.47083333 0.475 0.47916667 0.48333333 0.4875 0.49166667 0.49583333 0.5 0.50416667 0.50833333 0.5125 0.51666667 0.52083333 0.525 0.52916667 0.53333333 0.5375 0.54166667 0.54583333 0.55 0.55416667 0.55833333 0.5625 0.56666667 0.57083333 0.575 0.57916667 0.58333333 0.5875 0.59166667 0.59583333 0.6 0.60416667 0.60833333 0.6125 0.61666667 0.62083333 0.625 0.62916667 0.63333333 0.6375 0.64166667 0.64583333 0.65 0.65416667 0.65833333 0.6625 0.66666667 0.67083333 0.675 0.67916667 0.68333333 0.6875 0.69166667 0.69583333 0.7 0.70416667 0.70833333 0.7125 0.71666667 0.72083333 0.725 0.72916667 0.73333333 0.7375 0.74166667 0.74583333 0.75 0.75416667 0.75833333 0.7625 0.76666667 0.77083333 0.775 0.77916667 0.78333333 0.7875 0.79166667 0.79583333 0.8 0.80416667 0.80833333 0.8125 0.81666667 0.82083333 0.825 0.82916667 0.83333333 0.8375 0.84166667 0.84583333 0.85 0.85416667 0.85833333 0.8625 0.86666667 0.87083333 0.875 0.87916667 0.88333333 0.8875 0.89166667 0.89583333 0.9 0.90416667 0.90833333 0.9125 0.91666667 0.92083333 0.925 0.92916667 0.93333333 0.9375 0.94166667 0.94583333 0.95 0.95416667 0.95833333 0.9625 0.96666667 0.97083333 0.975 0.97916667 0.98333333 0.9875 0.99166667 0.99583333 1 1 1 1 1 1
  arc A9 (8.5381, -0.5989) -> (8.5381, 0.5989) centre (0, 0) ccw
  spline S9 degree 5 poles (8.5381, 0.5989) (8.5357, 0.6006) (8.5309, 0.604) (8.5237, 0.6091) (8.5141, 0.6158) (8.5021, 0.6241) (8.4901, 0.6324) (8.4782, 0.6406) (8.4662, 0.6488) (8.4542, 0.657) (8.4423, 0.665) (8.4303, 0.6731) (8.4184, 0.6811) (8.4064, 0.689) (8.3945, 0.6969) (8.3826, 0.7047) (8.3707, 0.7125) (8.3587, 0.7202) (8.3468, 0.7279) (8.3349, 0.7355) (8.3231, 0.743) (8.3112, 0.7506) (8.2993, 0.758) (8.2874, 0.7655) (8.2756, 0.7728) (8.2637, 0.7801) (8.2519, 0.7874) (8.2401, 0.7946) (8.2282, 0.8018) (8.2164, 0.8089) (8.2046, 0.8159) (8.1928, 0.8229) (8.1811, 0.8299) (8.1693, 0.8368) (8.1575, 0.8436) (8.1458, 0.8504) (8.1341, 0.8572) (8.1224, 0.8639) (8.1107, 0.8705) (8.099, 0.8771) (8.0873, 0.8837) (8.0756, 0.8902) (8.064, 0.8966) (8.0523, 0.903) (8.0407, 0.9094) (8.0291, 0.9157) (8.0175, 0.9219) (8.0059, 0.9281) (7.9943, 0.9342) (7.9828, 0.9403) (7.9713, 0.9464) (7.9597, 0.9524) (7.9482, 0.9583) (7.9368, 0.9642) (7.9253, 0.97) (7.9138, 0.9758) (7.9024, 0.9815) (7.891, 0.9872) (7.8796, 0.9929) (7.8682, 0.9985) (7.8569, 1.004) (7.8455, 1.0095) (7.8342, 1.0149) (7.8229, 1.0203) (7.8116, 1.0256) (7.8003, 1.0309) (7.7891, 1.0362) (7.7779, 1.0414) (7.7667, 1.0465) (7.7555, 1.0516) (7.7444, 1.0566) (7.7332, 1.0616) (7.7221, 1.0665) (7.711, 1.0714) (7.7, 1.0763) (7.6889, 1.0811) (7.6779, 1.0858) (7.6669, 1.0905) (7.6559, 1.0951) (7.645, 1.0997) (7.6341, 1.1043) (7.6232, 1.1088) (7.6123, 1.1132) (7.6014, 1.1176) (7.5906, 1.122) (7.5798, 1.1263) (7.5691, 1.1306) (7.5583, 1.1348) (7.5476, 1.1389) (7.5369, 1.143) (7.5263, 1.1471) (7.5157, 1.1511) (7.5051, 1.1551) (7.4945, 1.159) (7.4839, 1.1629) (7.4734, 1.1667) (7.463, 1.1705) (7.4525, 1.1742) (7.4421, 1.1779) (7.4317, 1.1815) (7.4214, 1.1851) (7.411, 1.1887) (7.4007, 1.1922) (7.3905, 1.1956) (7.3803, 1.199) (7.3701, 1.2024) (7.3599, 1.2057) (7.3498, 1.2089) (7.3397, 1.2122) (7.3296, 1.2153) (7.3196, 1.2185) (7.3096, 1.2215) (7.2997, 1.2246) (7.2898, 1.2276) (7.2799, 1.2305) (7.2701, 1.2334) (7.2603, 1.2363) (7.2505, 1.2391) (7.2408, 1.2419) (7.2311, 1.2446) (7.2215, 1.2473) (7.2118, 1.2499) (7.2023, 1.2525) (7.1928, 1.255) (7.1833, 1.2575) (7.1738, 1.26) (7.1644, 1.2624) (7.1551, 1.2648) (7.1457, 1.2671) (7.1365, 1.2694) (7.1272, 1.2717) (7.118, 1.2739) (7.1089, 1.276) (7.0998, 1.2782) (7.0907, 1.2802) (7.0817, 1.2823) (7.0728, 1.2843) (7.0638, 1.2862) (7.055, 1.2881) (7.0461, 1.29) (7.0374, 1.2918) (7.0286, 1.2936) (7.0199, 1.2954) (7.0113, 1.2971) (7.0027, 1.2988) (6.9942, 1.3004) (6.9857, 1.302) (6.9773, 1.3036) (6.9689, 1.3051) (6.9606, 1.3066) (6.9523, 1.308) (6.9441, 1.3094) (6.9359, 1.3108) (6.9278, 1.3121) (6.9197, 1.3134) (6.9117, 1.3146) (6.9037, 1.3159) (6.8958, 1.317) (6.888, 1.3182) (6.8802, 1.3193) (6.8725, 1.3204) (6.8648, 1.3214) (6.8572, 1.3224) (6.8496, 1.3234) (6.8421, 1.3243) (6.8347, 1.3252) (6.8273, 1.3261) (6.82, 1.3269) (6.8127, 1.3277) (6.8055, 1.3285) (6.7984, 1.3292) (6.7913, 1.3299) (6.7843, 1.3306) (6.7774, 1.3313) (6.7705, 1.3319) (6.7637, 1.3325) (6.7569, 1.333) (6.7503, 1.3335) (6.7437, 1.334) (6.7371, 1.3345) (6.7306, 1.3349) (6.7242, 1.3353) (6.7179, 1.3357) (6.7116, 1.3361) (6.7054, 1.3364) (6.6993, 1.3367) (6.6933, 1.337) (6.6873, 1.3372) (6.6814, 1.3374) (6.6755, 1.3376) (6.6698, 1.3378) (6.6641, 1.338) (6.6585, 1.3381) (6.653, 1.3382) (6.6475, 1.3383) (6.6422, 1.3383) (6.6369, 1.3384) (6.6317, 1.3384) (6.6265, 1.3384) (6.6215, 1.3384) (6.6165, 1.3383) (6.6117, 1.3383) (6.6069, 1.3382) (6.6021, 1.3381) (6.5975, 1.338) (6.593, 1.3379) (6.5885, 1.3377) (6.5842, 1.3376) (6.5799, 1.3374) (6.5757, 1.3372) (6.5716, 1.337) (6.5676, 1.3368) (6.5637, 1.3366) (6.5599, 1.3364) (6.5562, 1.3362) (6.5526, 1.3359) (6.549, 1.3357) (6.5456, 1.3354) (6.5423, 1.3352) (6.5391, 1.3349) (6.5359, 1.3346) (6.5329, 1.3343) (6.53, 1.3341) (6.5272, 1.3338) (6.5245, 1.3335) (6.5219, 1.3332) (6.5194, 1.3329) (6.517, 1.3326) (6.5147, 1.3324) (6.5126, 1.3321) (6.5105, 1.3318) (6.5086, 1.3316) (6.5068, 1.3313) (6.5051, 1.3311) (6.5035, 1.3308) (6.502, 1.3306) (6.5007, 1.3304) (6.4995, 1.3302) (6.4984, 1.33) (6.4975, 1.3299) (6.4966, 1.3297) (6.4961, 1.3296) (6.4957, 1.3295) (6.4955, 1.3295) (6.4954, 1.3295) knots -1 -1 -1 -1 -1 -1 -0.99583333 -0.99166667 -0.9875 -0.98333333 -0.97916667 -0.975 -0.97083333 -0.96666667 -0.9625 -0.95833333 -0.95416667 -0.95 -0.94583333 -0.94166667 -0.9375 -0.93333333 -0.92916667 -0.925 -0.92083333 -0.91666667 -0.9125 -0.90833333 -0.90416667 -0.9 -0.89583333 -0.89166667 -0.8875 -0.88333333 -0.87916667 -0.875 -0.87083333 -0.86666667 -0.8625 -0.85833333 -0.85416667 -0.85 -0.84583333 -0.84166667 -0.8375 -0.83333333 -0.82916667 -0.825 -0.82083333 -0.81666667 -0.8125 -0.80833333 -0.80416667 -0.8 -0.79583333 -0.79166667 -0.7875 -0.78333333 -0.77916667 -0.775 -0.77083333 -0.76666667 -0.7625 -0.75833333 -0.75416667 -0.75 -0.74583333 -0.74166667 -0.7375 -0.73333333 -0.72916667 -0.725 -0.72083333 -0.71666667 -0.7125 -0.70833333 -0.70416667 -0.7 -0.69583333 -0.69166667 -0.6875 -0.68333333 -0.67916667 -0.675 -0.67083333 -0.66666667 -0.6625 -0.65833333 -0.65416667 -0.65 -0.64583333 -0.64166667 -0.6375 -0.63333333 -0.62916667 -0.625 -0.62083333 -0.61666667 -0.6125 -0.60833333 -0.60416667 -0.6 -0.59583333 -0.59166667 -0.5875 -0.58333333 -0.57916667 -0.575 -0.57083333 -0.56666667 -0.5625 -0.55833333 -0.55416667 -0.55 -0.54583333 -0.54166667 -0.5375 -0.53333333 -0.52916667 -0.525 -0.52083333 -0.51666667 -0.5125 -0.50833333 -0.50416667 -0.5 -0.49583333 -0.49166667 -0.4875 -0.48333333 -0.47916667 -0.475 -0.47083333 -0.46666667 -0.4625 -0.45833333 -0.45416667 -0.45 -0.44583333 -0.44166667 -0.4375 -0.43333333 -0.42916667 -0.425 -0.42083333 -0.41666667 -0.4125 -0.40833333 -0.40416667 -0.4 -0.39583333 -0.39166667 -0.3875 -0.38333333 -0.37916667 -0.375 -0.37083333 -0.36666667 -0.3625 -0.35833333 -0.35416667 -0.35 -0.34583333 -0.34166667 -0.3375 -0.33333333 -0.32916667 -0.325 -0.32083333 -0.31666667 -0.3125 -0.30833333 -0.30416667 -0.3 -0.29583333 -0.29166667 -0.2875 -0.28333333 -0.27916667 -0.275 -0.27083333 -0.26666667 -0.2625 -0.25833333 -0.25416667 -0.25 -0.24583333 -0.24166667 -0.2375 -0.23333333 -0.22916667 -0.225 -0.22083333 -0.21666667 -0.2125 -0.20833333 -0.20416667 -0.2 -0.19583333 -0.19166667 -0.1875 -0.18333333 -0.17916667 -0.175 -0.17083333 -0.16666667 -0.1625 -0.15833333 -0.15416667 -0.15 -0.14583333 -0.14166667 -0.1375 -0.13333333 -0.12916667 -0.125 -0.12083333 -0.11666667 -0.1125 -0.10833333 -0.10416667 -0.1 -0.09583333 -0.09166667 -0.0875 -0.08333333 -0.07916667 -0.075 -0.07083333 -0.06666667 -0.0625 -0.05833333 -0.05416667 -0.05 -0.04583333 -0.04166667 -0.0375 -0.03333333 -0.02916667 -0.025 -0.02083333 -0.01666667 -0.0125 -0.00833333 -0.00416667 0 0 0 0 0 0
  line L18 (6.4954, 1.3295) -> (6.4945, 1.3293)
  line L19 (6.4945, 1.3293) -> (4.6119, 0.944)
  arc A10 (4.6119, 0.944) -> (3.9286, 2.5936) centre (0, 0) ccw
  line L20 (3.9286, 2.5936) -> (5.5323, 3.6523)
  line L21 (5.5323, 3.6523) -> (5.533, 3.6529)
  spline S10 degree 5 poles (5.533, 3.6529) (5.5331, 3.6529) (5.5333, 3.653) (5.5336, 3.6532) (5.5341, 3.6536) (5.5348, 3.654) (5.5355, 3.6546) (5.5364, 3.6552) (5.5374, 3.656) (5.5385, 3.6568) (5.5397, 3.6576) (5.541, 3.6586) (5.5424, 3.6596) (5.5438, 3.6607) (5.5454, 3.6619) (5.547, 3.6632) (5.5487, 3.6645) (5.5505, 3.6659) (5.5524, 3.6674) (5.5544, 3.6689) (5.5564, 3.6706) (5.5585, 3.6723) (5.5607, 3.6741) (5.563, 3.676) (5.5653, 3.6779) (5.5677, 3.6799) (5.5702, 3.682) (5.5727, 3.6842) (5.5753, 3.6864) (5.578, 3.6887) (5.5807, 3.6911) (5.5835, 3.6936) (5.5864, 3.6961) (5.5893, 3.6987) (5.5923, 3.7014) (5.5953, 3.7042) (5.5984, 3.707) (5.6015, 3.7099) (5.6047, 3.7129) (5.608, 3.7159) (5.6113, 3.719) (5.6146, 3.7222) (5.618, 3.7255) (5.6214, 3.7288) (5.6249, 3.7323) (5.6285, 3.7357) (5.6321, 3.7393) (5.6357, 3.7429) (5.6394, 3.7466) (5.6431, 3.7504) (5.6468, 3.7542) (5.6506, 3.7581) (5.6544, 3.7621) (5.6583, 3.7662) (5.6622, 3.7703) (5.6662, 3.7745) (5.6702, 3.7787) (5.6742, 3.7831) (5.6782, 3.7875) (5.6823, 3.7919) (5.6864, 3.7965) (5.6906, 3.8011) (5.6948, 3.8058) (5.699, 3.8105) (5.7032, 3.8153) (5.7075, 3.8202) (5.7118, 3.8252) (5.7161, 3.8302) (5.7205, 3.8353) (5.7248, 3.8405) (5.7292, 3.8457) (5.7337, 3.851) (5.7381, 3.8563) (5.7426, 3.8618) (5.7471, 3.8673) (5.7516, 3.8728) (5.7562, 3.8785) (5.7607, 3.8842) (5.7653, 3.8899) (5.7699, 3.8958) (5.7745, 3.9017) (5.7792, 3.9076) (5.7838, 3.9137) (5.7885, 3.9198) (5.7932, 3.9259) (5.7979, 3.9321) (5.8026, 3.9384) (5.8074, 3.9448) (5.8121, 3.9512) (5.8169, 3.9577) (5.8217, 3.9643) (5.8265, 3.9709) (5.8313, 3.9776) (5.8361, 3.9843) (5.8409, 3.9911) (5.8457, 3.998) (5.8506, 4.0049) (5.8554, 4.0119) (5.8603, 4.019) (5.8652, 4.0261) (5.8701, 4.0333) (5.8749, 4.0406) (5.8798, 4.0479) (5.8847, 4.0553) (5.8896, 4.0627) (5.8945, 4.0702) (5.8995, 4.0778) (5.9044, 4.0854) (5.9093, 4.0931) (5.9142, 4.1008) (5.9192, 4.1086) (5.9241, 4.1165) (5.929, 4.1245) (5.934, 4.1325) (5.9389, 4.1405) (5.9439, 4.1486) (5.9488, 4.1568) (5.9537, 4.165) (5.9587, 4.1733) (5.9636, 4.1817) (5.9686, 4.1901) (5.9735, 4.1986) (5.9784, 4.2071) (5.9834, 4.2157) (5.9883, 4.2244) (5.9932, 4.2331) (5.9981, 4.2419) (6.0031, 4.2507) (6.008, 4.2596) (6.0129, 4.2686) (6.0178, 4.2776) (6.0227, 4.2866) (6.0276, 4.2958) (6.0325, 4.3049) (6.0373, 4.3142) (6.0422, 4.3235) (6.0471, 4.3328) (6.0519, 4.3422) (6.0568, 4.3517) (6.0616, 4.3612) (6.0665, 4.3708) (6.0713, 4.3804) (6.0761, 4.3901) (6.0809, 4.3999) (6.0857, 4.4097) (6.0905, 4.4195) (6.0952, 4.4295) (6.1, 4.4394) (6.1048, 4.4495) (6.1095, 4.4595) (6.1142, 4.4697) (6.1189, 4.4799) (6.1236, 4.4901) (6.1283, 4.5004) (6.133, 4.5108) (6.1377, 4.5212) (6.1423, 4.5316) (6.1469, 4.5421) (6.1516, 4.5527) (6.1562, 4.5633) (6.1607, 4.574) (6.1653, 4.5847) (6.1699, 4.5955) (6.1744, 4.6064) (6.1789, 4.6172) (6.1835, 4.6282) (6.1879, 4.6392) (6.1924, 4.6502) (6.1969, 4.6613) (6.2013, 4.6725) (6.2057, 4.6836) (6.2101, 4.6949) (6.2145, 4.7062) (6.2189, 4.7175) (6.2232, 4.7289) (6.2275, 4.7404) (6.2319, 4.7519) (6.2361, 4.7634) (6.2404, 4.7751) (6.2447, 4.7867) (6.2489, 4.7984) (6.2531, 4.8102) (6.2573, 4.822) (6.2614, 4.8338) (6.2656, 4.8457) (6.2697, 4.8577) (6.2738, 4.8696) (6.2779, 4.8817) (6.2819, 4.8938) (6.2859, 4.9059) (6.2899, 4.9181) (6.2939, 4.9304) (6.2979, 4.9426) (6.3018, 4.955) (6.3057, 4.9673) (6.3096, 4.9798) (6.3135, 4.9922) (6.3173, 5.0048) (6.3211, 5.0173) (6.3249, 5.0299) (6.3287, 5.0426) (6.3324, 5.0553) (6.3361, 5.0681) (6.3398, 5.0809) (6.3434, 5.0937) (6.3471, 5.1066) (6.3507, 5.1195) (6.3542, 5.1325) (6.3578, 5.1455) (6.3613, 5.1586) (6.3648, 5.1717) (6.3683, 5.1849) (6.3717, 5.1981) (6.3751, 5.2113) (6.3785, 5.2246) (6.3819, 5.2379) (6.3852, 5.2513) (6.3885, 5.2647) (6.3917, 5.2782) (6.395, 5.2917) (6.3982, 5.3053) (6.4014, 5.3188) (6.4045, 5.3325) (6.4076, 5.3462) (6.4107, 5.3599) (6.4138, 5.3736) (6.4168, 5.3874) (6.4198, 5.4013) (6.4227, 5.4152) (6.4257, 5.4291) (6.4286, 5.4431) (6.4314, 5.4571) (6.4343, 5.4711) (6.4371, 5.4852) (6.4399, 5.4993) (6.4426, 5.5135) (6.4453, 5.5277) (6.448, 5.542) (6.4506, 5.5563) (6.4532, 5.5706) (6.4558, 5.585) (6.4578, 5.5965) (6.4593, 5.6051) (6.4603, 5.6109) (6.4608, 5.6138) knots 0 0 0 0 0 0 0.00416667 0.00833333 0.0125 0.01666667 0.02083333 0.025 0.02916667 0.03333333 0.0375 0.04166667 0.04583333 0.05 0.05416667 0.05833333 0.0625 0.06666667 0.07083333 0.075 0.07916667 0.08333333 0.0875 0.09166667 0.09583333 0.1 0.10416667 0.10833333 0.1125 0.11666667 0.12083333 0.125 0.12916667 0.13333333 0.1375 0.14166667 0.14583333 0.15 0.15416667 0.15833333 0.1625 0.16666667 0.17083333 0.175 0.17916667 0.18333333 0.1875 0.19166667 0.19583333 0.2 0.20416667 0.20833333 0.2125 0.21666667 0.22083333 0.225 0.22916667 0.23333333 0.2375 0.24166667 0.24583333 0.25 0.25416667 0.25833333 0.2625 0.26666667 0.27083333 0.275 0.27916667 0.28333333 0.2875 0.29166667 0.29583333 0.3 0.30416667 0.30833333 0.3125 0.31666667 0.32083333 0.325 0.32916667 0.33333333 0.3375 0.34166667 0.34583333 0.35 0.35416667 0.35833333 0.3625 0.36666667 0.37083333 0.375 0.37916667 0.38333333 0.3875 0.39166667 0.39583333 0.4 0.40416667 0.40833333 0.4125 0.41666667 0.42083333 0.425 0.42916667 0.43333333 0.4375 0.44166667 0.44583333 0.45 0.45416667 0.45833333 0.4625 0.46666667 0.47083333 0.475 0.47916667 0.48333333 0.4875 0.49166667 0.49583333 0.5 0.50416667 0.50833333 0.5125 0.51666667 0.52083333 0.525 0.52916667 0.53333333 0.5375 0.54166667 0.54583333 0.55 0.55416667 0.55833333 0.5625 0.56666667 0.57083333 0.575 0.57916667 0.58333333 0.5875 0.59166667 0.59583333 0.6 0.60416667 0.60833333 0.6125 0.61666667 0.62083333 0.625 0.62916667 0.63333333 0.6375 0.64166667 0.64583333 0.65 0.65416667 0.65833333 0.6625 0.66666667 0.67083333 0.675 0.67916667 0.68333333 0.6875 0.69166667 0.69583333 0.7 0.70416667 0.70833333 0.7125 0.71666667 0.72083333 0.725 0.72916667 0.73333333 0.7375 0.74166667 0.74583333 0.75 0.75416667 0.75833333 0.7625 0.76666667 0.77083333 0.775 0.77916667 0.78333333 0.7875 0.79166667 0.79583333 0.8 0.80416667 0.80833333 0.8125 0.81666667 0.82083333 0.825 0.82916667 0.83333333 0.8375 0.84166667 0.84583333 0.85 0.85416667 0.85833333 0.8625 0.86666667 0.87083333 0.875 0.87916667 0.88333333 0.8875 0.89166667 0.89583333 0.9 0.90416667 0.90833333 0.9125 0.91666667 0.92083333 0.925 0.92916667 0.93333333 0.9375 0.94166667 0.94583333 0.95 0.95416667 0.95833333 0.9625 0.96666667 0.97083333 0.975 0.97916667 0.98333333 0.9875 0.99166667 0.99583333 1 1 1 1 1 1
  arc A11 (6.4608, 5.6138) -> (5.6138, 6.4608) centre (0, 0) ccw